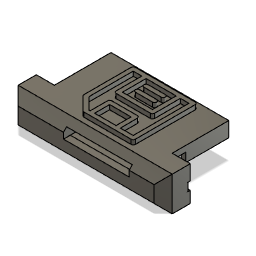
SD Module Cover Plate (Autodesk Fusion 360 design; units mm, degrees)
Autodesk Fusion 360 part; units mm, degrees
note: some values were not read from the file. Set by a fixed rule: which sketch regions a step uses.
sketch "Sketch1" plane through (0, 0, 0) normal (0, 1, 0) x (1, 0, 0)
  line L0 (0, 0) -> (0, 17)
  line L1 (0, 0) -> (0, -1.5)
  line L2 (0, -1.5) -> (26, -1.5)
  line L3 (26, -1.5) -> (26, 17)
  line L4 (26, 17) -> (0, 17)
  dimension "d2" = 17
  dimension "d3" = 1.5
  dimension "d5" = 26
  constraint coincident L0.start L1.start
  constraint perpendicular L1 L2
  constraint perpendicular L2 L3
  constraint coincident L0.end L4.end
  constraint vertical L3
  constraint horizontal L4
  constraint vertical L0
  measures "d2" distance of L0.start L0.end
  measures "d3" distance of L0.start L1.end
  measures "d5" horizontal distance of L1.end L2.end
extrude "Extrude1" add sketch "Sketch1" along normal blind 3.3
sketch "Sketch2" plane through (0, 0, 0) normal (0, -1, 0) x (1, 0, 0)
  line L0 (0, 1.5) -> (0, -17)
  line L1 (0, -17) -> (26, -17)
  line L2 (26, -17) -> (26, 1.5)
  line L3 (26, 1.5) -> (0, 1.5)
  line L4 (25, -0.5) -> (25, -3.5)
  line L5 (25, -3.5) -> (26, -3.5)
  line L6 (26, -7.5) -> (25, -7.5)
  line L7 (25, -7.5) -> (25, -17)
  line L8 (25, -17) -> (2, -17)
  line L9 (2, -17) -> (2, -7.5)
  line L10 (2, -7.5) -> (8, -7.5)
  line L11 (8, -7.5) -> (8, 1.5)
  line L12 (25, -0.5) -> (22.5, -0.5)
  line L13 (22.5, -0.5) -> (22.5, 1.5)
  dimension "d9" = 2
  dimension "d10" = 1
  dimension "d11" = 3.5
  dimension "d12" = 8
  dimension "d14" = 3
  dimension "d15" = 4
  dimension "d16" = 2
  dimension "d17" = 7
  constraint perpendicular L3 L4
  constraint coincident L2 L5.end
  constraint coincident L2 L6.start
  constraint perpendicular L2 L6
  constraint perpendicular L6 L7
  constraint perpendicular L2 L8
  constraint perpendicular L1 L9
  constraint perpendicular L9 L10
  constraint coincident L3 L11.end
  constraint perpendicular L4 L12
  constraint coincident L3 L13.end
  constraint collinear L4 L7
  constraint collinear L1 L8
  measures "d9" distance of L0 L9
  measures "d10" distance of L2 L4
  measures "d11" distance of L2 L13
  measures "d12" distance of L0 L11
  measures "d14" distance of L5 L12
  measures "d15" distance of L5 L6
  measures "d16" distance of L3 L12
  measures "d17" distance of L10 L12
extrude "Extrude3" cut sketch "Sketch2" against normal blind 2 contours L1 L2 L3 L4 L5 L6 L7 L8 L9 L10 L11 L12 L13
sketch "Sketch3" plane through (13, 0, -8.75) normal (0, -1, 0) x (1, 0, 0)
  line L0 (-13, 10.25) -> (13, 10.25)
  line L1 (13, 10.25) -> (13, 8.75)
  line L2 (13, 8.75) -> (-13, 8.75)
  line L3 (-13, 8.75) -> (-13, 10.25)
  line L4 (13, 10.25) -> (13, 5.25)
  line L5 (13, 10.25) -> (13, -8.25)
  line L6 (13, -8.25) -> (13, 10.25)
  point P0 (-13, 10.25)
  dimension "d22" = 1.5
  constraint horizontal L0
  constraint vertical L1
  constraint horizontal L2
  constraint vertical L3
  constraint coincident L1.end L4
  constraint coincident P0 L0.start
  measures "d22" distance of L0 L2
extrude "Extrude4" add sketch "Sketch3" along normal blind 1.8
sketch "Sketch4" plane through (0, -1.8, 0) normal (0, -1, 0) x (1, 0, 0)
  line L0 (26, 0) -> (26, 1.5)
  line L1 (26, 1.5) -> (0, 1.5)
  line L2 (0, 1.5) -> (0, 0)
  line L3 (0, 0) -> (26, 0)
  line L4 (26, 1.5) -> (0, 1.5)
  line L5 (0, 1.5) -> (0, -6.5)
  line L6 (0, -6.5) -> (26, -6.5)
  line L7 (26, -6.5) -> (26, 1.5)
  line L8 (0, 1.5) -> (0, 0)
  dimension "d25" = 8
  constraint horizontal L4
  constraint vertical L5
  constraint horizontal L6
  constraint vertical L7
  constraint coincident L0.end L1.start
  constraint collinear L5 L8
  measures "d25" vertical distance of L1.end L5.end
extrude "Extrude5" add sketch "Sketch4" along normal blind 2.5
sketch "Sketch5" plane through (0, 3.3, 0) normal (0, 1, 0) x (-1, 0, 0)
  line L0 (0, -17) -> (0, 1.5)
  line L1 (0, 1.5) -> (-26, 1.5)
  line L2 (-26, 1.5) -> (-26, -17)
  line L3 (-26, -17) -> (0, -17)
  line L4 (-26, 1.5) -> (-30, 1.5)
  line L5 (-30, 1.5) -> (-30, -4.5)
  line L6 (-30, -4.5) -> (-26, -4.5)
  line L7 (-26, -4.5) -> (-26, 1.5)
  line L8 (-26, 0) -> (-22.5, 0)
  line L9 (-26, 0) -> (-30.5, -4.5)
  line L10 (-13, 15.8089) -> (-13, -12.8089) construction
  line L11 (0, 1.5) -> (4, 1.5)
  line L12 (4, 1.5) -> (4, -4.5)
  line L13 (4, -4.5) -> (0, -4.5)
  line L14 (0, 0) -> (4.5, -4.5)
  line L15 (0, -4.5) -> (0, 1.5)
  dimension "d28" = 45
  dimension "d29" = 4
  dimension "d30" = 6
  constraint horizontal L4
  constraint vertical L5
  constraint horizontal L6
  constraint vertical L7
  constraint coincident L1.end L2.start
  constraint coincident L8.start L9.start
  constraint coincident L6 L9.end
  constraint vertical L10
  constraint midpoint L1 L10
  constraint symmetric L1.end L10 L0.end
  constraint symmetric L4.end L10 L11.end
  constraint symmetric L5.end L10 L12.end
  constraint symmetric L6.end L10 L13.end
  constraint symmetric L8.start L10 L14.start
  constraint symmetric L9.end L10 L14.end
  measures "d28" angle of L7 L9
  measures "d29" distance of L1.end L4.end
  measures "d30" distance of L4.end L5.end
extrude "Extrude6" add sketch "Sketch5" against normal up to surface (7.6 mm away) contours L0 L12 L13 L14 L15 | L0 L11 L12 L14 L15 | L2 L5 L6 L7 L9 | L2 L4 L5 L7 L9
extrude "Extrude7" cut sketch "Sketch5" against normal up to surface (1.8 mm away) from surface at -3.3 contours L0 L12 L13 L14 L15 | L2 L5 L6 L7 L9
chamfer "Chamfer1" distance 2 angle 45 4 edges at (-4, -0.5, 1.5) (13, 3.3, 1.5) (30, -0.5, 1.5) (13, -4.3, 1.5)
sketch "Sketch7" plane through (0, 3.3, 0) normal (0, 1, 0) x (-1, 0, 0)
  line L0 (4, -0.5) -> (-30, -0.5)
  line L1 (-30, -0.5) -> (-30, -4.5)
  line L2 (-30, -4.5) -> (-26, -4.5)
  line L3 (-26, -4.5) -> (-26, -17)
  line L4 (-26, -17) -> (0, -17)
  line L5 (0, -17) -> (0, -4.5)
  line L6 (0, -4.5) -> (4, -4.5)
  line L7 (4, -4.5) -> (4, -0.5)
  arc A0 (-9.3674, -1.646) -> (-9.0314, -1.7832) centre (-9.3647, -2.1193) cw
  line L8 (-9.3674, -1.646) -> (-19.7793, -1.646)
  arc A1 (-20.2526, -2.1193) -> (-19.7793, -1.646) centre (-19.7793, -2.1193) cw
  line L9 (-20.2526, -2.1193) -> (-20.2526, -15.3708)
  arc A2 (-19.7793, -15.8441) -> (-20.2526, -15.3708) centre (-19.7793, -15.3708) cw
  line L10 (-19.7793, -15.8441) -> (-6.5278, -15.8441)
  arc A3 (-6.0545, -15.3708) -> (-6.5278, -15.8441) centre (-6.5278, -15.3708) cw
  line L11 (-6.0545, -15.3708) -> (-6.0545, -4.9589)
  arc A4 (-6.1918, -4.6229) -> (-6.0545, -4.9589) centre (-6.5278, -4.9561) cw
  line L12 (-6.1918, -4.6229) -> (-9.0314, -1.7832)
  line L13 (-10.7872, -2.5925) -> (-10.7872, -5.9054)
  line L14 (-10.7872, -5.9054) -> (-15.5199, -5.9054)
  line L15 (-15.5199, -5.9054) -> (-15.5199, -2.5925)
  line L16 (-15.5199, -2.5925) -> (-10.7872, -2.5925)
  line L17 (-16.4664, -14.8975) -> (-16.4664, -9.6916)
  line L18 (-16.4664, -9.6916) -> (-9.8407, -9.6916)
  line L19 (-9.8407, -9.6916) -> (-9.8407, -14.8975)
  line L20 (-9.8407, -14.8975) -> (-16.4664, -14.8975)
  line L21 (-7.0011, -14.8975) -> (-8.8941, -14.8975)
  line L22 (-8.8941, -14.8975) -> (-8.8941, -9.2183)
  arc A5 (-9.3674, -8.745) -> (-8.8941, -9.2183) centre (-9.3674, -9.2183) cw
  line L23 (-9.3674, -8.745) -> (-16.9397, -8.745)
  arc A6 (-17.413, -9.2183) -> (-16.9397, -8.745) centre (-16.9397, -9.2183) cw
  line L24 (-17.413, -9.2183) -> (-17.413, -14.8975)
  line L25 (-17.413, -14.8975) -> (-19.306, -14.8975)
  line L26 (-19.306, -14.8975) -> (-19.306, -2.5925)
  line L27 (-19.306, -2.5925) -> (-16.4664, -2.5925)
  line L28 (-16.4664, -2.5925) -> (-16.4664, -6.3787)
  arc A7 (-15.9932, -6.8519) -> (-16.4664, -6.3787) centre (-15.9932, -6.3787) cw
  line L29 (-15.9932, -6.8519) -> (-10.3139, -6.8519)
  arc A8 (-9.8407, -6.3787) -> (-10.3139, -6.8519) centre (-10.3139, -6.3787) cw
  line L30 (-9.8407, -6.3787) -> (-9.8407, -2.5925)
  line L31 (-9.8407, -2.5925) -> (-9.5614, -2.5925)
  line L32 (-9.5614, -2.5925) -> (-7.0011, -5.1529)
  line L33 (-7.0011, -5.1529) -> (-7.0011, -14.8975)
  line L34 (-11.2605, -11.1114) -> (-15.0466, -11.1114)
  arc A9 (-15.0466, -12.0579) -> (-15.0466, -11.1114) centre (-15.0466, -11.5846) cw
  line L35 (-15.0466, -12.0579) -> (-11.2605, -12.0579)
  arc A10 (-11.2605, -11.1114) -> (-11.2605, -12.0579) centre (-11.2605, -11.5846) cw
  line L36 (-11.2605, -13.0044) -> (-15.0466, -13.0044)
  arc A11 (-15.0466, -13.951) -> (-15.0466, -13.0044) centre (-15.0466, -13.4777) cw
  line L37 (-15.0466, -13.951) -> (-11.2605, -13.951)
  arc A12 (-11.2605, -13.0044) -> (-11.2605, -13.951) centre (-11.2605, -13.4777) cw
extrude "Extrude9" add sketch "Sketch7" along normal blind 1 contours A0 L8 A1 L9 A2 L10 A3 L11 A4 L12 | L34 A9 L35 A10 | L36 A11 L37 A12
equation "d30 = 3.5 mm + 2.5 mm"
